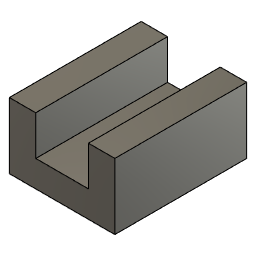
Connerctor v4 (Autodesk Fusion 360 design; units mm, degrees)
Autodesk Fusion 360 part; units mm, degrees
sketch "Sketch1" plane through (0, 0, 0) normal (0, 1, 0) x (1, 0, 0)
  line L0 (0, 0) -> (8, 0)
  line L1 (8, 0) -> (8, 10)
  line L2 (8, 10) -> (0, 10)
  line L3 (0, 10) -> (0, 0)
  dimension "d1" = 8
  dimension "d2" = 10
  constraint horizontal L0
  constraint vertical L1
  constraint horizontal L2
  constraint vertical L3
  constraint coincident L0.start L3.end
  measures "d1" distance of L0.start L0.end
  measures "d2" distance of L0.start L2.end
extrude "Extrude1" add sketch "Sketch1" along normal blind 2
sketch "Sketch3" plane through (0, 2, 0) normal (0, 1, 0) x (-1, 0, 0)
  line L0 (0, -10) -> (0, 0)
  line L1 (0, 0) -> (-8, 0)
  line L2 (-8, 0) -> (-8, -10)
  line L3 (-8, -10) -> (0, -10)
  line L4 (0, 0) -> (-2, 0)
  line L5 (-2, 0) -> (-2, -10)
  line L6 (-2, -10) -> (0, -10)
  line L7 (0, -10) -> (0, 0)
  line L8 (-8, 0) -> (-6, 0)
  line L9 (-6, 0) -> (-6, -10)
  line L10 (-6, -10) -> (-8, -10)
  line L11 (-8, -10) -> (-8, 0)
  dimension "d5" = 2
  dimension "d6" = 2
  constraint horizontal L4
  constraint vertical L5
  constraint horizontal L6
  constraint vertical L7
  constraint coincident L3 L5.end
  constraint coincident L0.end L1.start
  constraint horizontal L8
  constraint vertical L9
  constraint horizontal L10
  constraint vertical L11
  constraint coincident L3 L9.end
  constraint coincident L1.end L2.start
  measures "d5" distance of L0.end L4.end
  measures "d6" distance of L1.end L8.end
extrude "Extrude2" add sketch "Sketch3" along normal blind 3 contours L0 L1 L3 L4 L5 L6 L7 | L1 L2 L3 L8 L9 L10 L11
